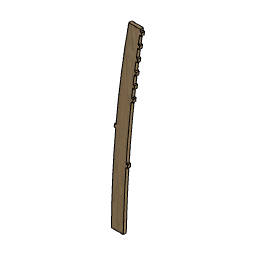
fotur_b (Autodesk Fusion 360 design; units mm, degrees)
Autodesk Fusion 360 part; units mm, degrees
note: some values were not read from the file. Set by a fixed rule: which sketch regions a step uses.
sketch "Sketch1" plane through (0, 0, 0) normal (0, 1, 0) x (1, 0, 0)
  line L0 (0, 0) -> (175, 0)
  line L1 (175, 0) -> (175, -1200)
  line L2 (175, -1200) -> (0, -1200)
  line L3 (0, -1200) -> (0, 0)
  line L4 (0, 0) -> (70, 0)
  line L5 (0, -1200) -> (0, -600)
  arc A0 (70, 0) -> (175, -1200) centre (8172.5, 104.375) ccw
  line L6 (175, -1200) -> (105, -1200)
  arc A1 (0, 0) -> (105, -1200) centre (6634.3619, -24.0871) ccw
  dimension "d1" = 175
  dimension "d2" = 1200
  dimension "d3" = 70
  dimension "d7" = 600
  dimension "d9" = 70
  constraint horizontal L0
  constraint vertical L1
  constraint horizontal L2
  constraint vertical L3
  constraint coincident L0.start L3.end
  constraint perpendicular L3 L4
  constraint perpendicular L2 L5
  constraint perpendicular L1 L6
  measures "d1" distance of L0.start L0.end
  measures "d2" distance of L0.start L2.end
  measures "d3" distance of L0.start L4.end
  measures "d7" distance of L2.end L5.end
  measures "d9" distance of L1.end L6.end
extrude "Extrude1" add sketch "Sketch1" along normal blind 18 contours L0 L2 L3 L4 A0 L6 A1
sketch "Sketch2" plane through (0, 0, 0) normal (0, -1, 0) x (1, 0, 0)
  line L0 (0, 48.1742) -> (0, 0)
  line L1 (0, 0) -> (70, 0)
  arc A0 (175, 1200) -> (70, 0) centre (8172.5, -104.375) ccw
  line L2 (175, 1200) -> (105, 1200)
  arc A1 (105, 1200) -> (0, 48.1742) centre (6634.3619, 24.0871) ccw
  line L3 (172.5991, 1185.1934) -> (181.4831, 1183.7529)
  line L4 (181.4831, 1183.7529) -> (178.282, 1164.0107)
  line L5 (178.282, 1164.0107) -> (169.398, 1165.4512)
  line L6 (172.5991, 1185.1934) -> (169.398, 1165.4512)
  line L7 (150.1002, 1036.8969) -> (159.0061, 1035.5991)
  line L8 (159.0061, 1035.5991) -> (156.1221, 1015.8081)
  line L9 (156.1221, 1015.8081) -> (147.2161, 1017.1059)
  line L10 (139.8807, 962.5964) -> (148.7983, 961.381)
  line L11 (148.7983, 961.381) -> (146.0975, 941.5642)
  line L12 (146.0975, 941.5642) -> (137.18, 942.7795)
  line L13 (130.3495, 888.2053) -> (139.2798, 887.0876)
  line L14 (139.2798, 887.0876) -> (136.796, 867.2424)
  line L15 (136.796, 867.2424) -> (127.8657, 868.3602)
  line L16 (121.5072, 813.729) -> (130.4468, 812.6885)
  line L17 (130.4468, 812.6885) -> (128.1346, 792.8226)
  line L18 (128.1346, 792.8226) -> (119.195, 793.8631)
  line L19 (161.0062, 1111.0952) -> (169.9008, 1109.722)
  line L20 (169.9008, 1109.722) -> (166.8493, 1089.9562)
  line L21 (166.8493, 1089.9562) -> (157.9434, 1091.254)
  dimension "d15" = 15
  dimension "d17" = 9
  dimension "d18" = 20
  dimension "d19" = 9
  dimension "d29" = 9
  dimension "d30" = 20
  dimension "d31" = 9
  dimension "d33" = 9
  dimension "d34" = 20
  dimension "d35" = 9
  dimension "d40" = 55
  dimension "d41" = 9
  dimension "d42" = 20
  dimension "d43" = 9
  dimension "d44" = 55
  dimension "d45" = 9
  dimension "d46" = 20
  dimension "d47" = 9
  dimension "d48" = 55
  dimension "d49" = 9
  dimension "d50" = 20
  dimension "d51" = 9
  constraint perpendicular L3 L4
  constraint perpendicular L4 L5
  constraint coincident A0 L7.start
  constraint perpendicular L7 L8
  constraint perpendicular L8 L9
  constraint coincident A0 L10.start
  constraint perpendicular L10 L11
  constraint perpendicular L11 L12
  constraint coincident A0 L13.start
  constraint perpendicular L13 L14
  constraint perpendicular L14 L15
  constraint coincident A0 L16.start
  constraint perpendicular L16 L17
  constraint perpendicular L17 L18
  constraint coincident A0 L3.start
  constraint coincident A0 L19.start
  constraint perpendicular L19 L20
  measures "d15" distance of A0.start L3.start
  measures "d17" distance of L3.start L3.end
  measures "d18" distance of L3.end L4.end
  measures "d19" distance of L4.end L5.end
  measures "d29" distance of L7.start L7.end
  measures "d30" distance of L7.end L8.end
  measures "d31" distance of L8.end L9.end
  measures "d33" distance of L10.start L10.end
  measures "d34" distance of L10.end L11.end
  measures "d35" distance of L11.end L12.end
  measures "d40" distance of L12.end L13.start
  measures "d41" distance of L13.start L13.end
  measures "d42" distance of L13.end L14.end
  measures "d43" distance of L14.end L15.end
  measures "d44" distance of L15.end L16.start
  measures "d45" distance of L16.start L16.end
  measures "d46" distance of L16.end L17.end
  measures "d47" distance of L17.end L18.end
  measures "d48" distance of L5.end L19.start
  measures "d49" distance of L19.start L19.end
  measures "d50" distance of L19.end L20.end
  measures "d51" distance of L20.end L21.end
extrude "Extrude2" add sketch "Sketch2" against normal blind 18 contours A0 L16 L17 L18 | A0 L3 L4 L5 | A0 L5 L6 | A0 L13 L14 L15 | A0 L19 L20 L21 | A0 L10 L11 L12 | A0 L7 L8 L9
sketch "Sketch3" plane through (0, 0, 0) normal (0, -1, 0) x (1, 0, 0)
  arc A0 (175, 1200) -> (172.5991, 1185.1934) centre (8172.5, -104.375) ccw
  line L0 (175, 1200) -> (105, 1200)
  arc A1 (105, 1200) -> (0, 48.1742) centre (6634.3619, 24.0871) ccw
  line L1 (0, 48.1742) -> (0, 0)
  line L2 (0, 0) -> (70, 0)
  arc A2 (119.2656, 793.8548) -> (70, 0) centre (8172.5, -104.375) ccw
  line L3 (119.2656, 793.8548) -> (128.1346, 792.8226)
  line L4 (128.1346, 792.8226) -> (130.4468, 812.6885)
  line L5 (130.4468, 812.6885) -> (121.5072, 813.729)
  arc A3 (127.9241, 868.3528) -> (121.5072, 813.729) centre (8172.5, -104.375) ccw
  line L6 (127.9241, 868.3528) -> (136.796, 867.2424)
  line L7 (136.796, 867.2424) -> (139.2798, 887.0876)
  line L8 (139.2798, 887.0876) -> (130.3495, 888.2053)
  arc A4 (137.2717, 942.767) -> (130.3495, 888.2053) centre (8172.5, -104.375) ccw
  line L9 (137.2717, 942.767) -> (146.0975, 941.5642)
  line L10 (146.0975, 941.5642) -> (148.7983, 961.381)
  line L11 (148.7983, 961.381) -> (139.8807, 962.5964)
  arc A5 (147.3077, 1017.0926) -> (139.8807, 962.5964) centre (8172.5, -104.375) ccw
  line L12 (147.3077, 1017.0926) -> (156.1221, 1015.8081)
  line L13 (156.1221, 1015.8081) -> (159.0061, 1035.5991)
  line L14 (159.0061, 1035.5991) -> (150.1002, 1036.8969)
  line L15 (158.0195, 1091.2429) -> (166.8493, 1089.9562)
  line L16 (166.8493, 1089.9562) -> (169.9008, 1109.722)
  line L17 (169.9008, 1109.722) -> (161.0062, 1111.0952)
  arc A6 (169.4406, 1165.4443) -> (161.0062, 1111.0952) centre (8172.5, -104.375) ccw
  line L18 (169.4406, 1165.4443) -> (178.282, 1164.0107)
  line L19 (178.282, 1164.0107) -> (181.4831, 1183.7529)
  line L20 (181.4831, 1183.7529) -> (172.5991, 1185.1934)
  line L21 (88.6743, 455.2339) -> (97.6378, 454.4241)
  line L22 (97.6378, 454.4241) -> (95.8383, 434.5052)
  line L23 (95.8383, 434.5052) -> (86.8748, 435.315)
  line L24 (27.8153, 631.4419) -> (18.8644, 632.3806)
  line L25 (18.8644, 632.3806) -> (16.7784, 612.4897)
  line L26 (16.7784, 612.4897) -> (26.7239, 611.4467)
  dimension "d56" = 9
  dimension "d57" = 20
  dimension "d58" = 9
  dimension "d72" = 9
  dimension "d73" = 20
  dimension "d74" = 10
  constraint coincident A2 L21.start
  constraint perpendicular L21 L22
  constraint perpendicular L22 L23
  constraint coincident A1 L24.start
  constraint perpendicular L24 L25
  constraint perpendicular L25 L26
  measures "d56" distance of L21.start L21.end
  measures "d57" distance of L21.end L22.end
  measures "d58" distance of L22.end L23.end
  measures "d72" distance of L24.start L24.end
  measures "d73" distance of L24.end L25.end
  measures "d74" distance of L25.end L26.end
extrude "Extrude3" add sketch "Sketch3" against normal blind 18
sketch "Sketch4" plane through (0, 0, 0) normal (0, -1, 0) x (1, 0, 0)
  arc A0 (175, 1200) -> (172.5991, 1185.1934) centre (8172.5, -104.375) ccw
  line L0 (175, 1200) -> (105, 1200)
  arc A1 (105, 1200) -> (27.8153, 631.4419) centre (6634.3619, 24.0871) ccw
  line L1 (27.8153, 631.4419) -> (18.8644, 632.3806)
  line L2 (18.8644, 632.3806) -> (16.7784, 612.4897)
  line L3 (16.7784, 612.4897) -> (26.0142, 611.5211)
  arc A2 (26.0142, 611.5211) -> (0, 48.1742) centre (6634.3619, 24.0871) ccw
  line L4 (0, 48.1742) -> (0, 0)
  line L5 (0, 0) -> (70, 0)
  arc A3 (87.3174, 435.275) -> (70, 0) centre (8172.5, -104.375) ccw
  line L6 (87.3174, 435.275) -> (95.8383, 434.5052)
  line L7 (95.8383, 434.5052) -> (97.6378, 454.4241)
  line L8 (97.6378, 454.4241) -> (88.6743, 455.2339)
  arc A4 (119.2656, 793.8548) -> (88.6743, 455.2339) centre (8172.5, -104.375) ccw
  line L9 (119.2656, 793.8548) -> (128.1346, 792.8226)
  line L10 (128.1346, 792.8226) -> (130.4468, 812.6885)
  line L11 (130.4468, 812.6885) -> (121.5072, 813.729)
  arc A5 (127.9241, 868.3528) -> (121.5072, 813.729) centre (8172.5, -104.375) ccw
  line L12 (127.9241, 868.3528) -> (136.796, 867.2424)
  line L13 (136.796, 867.2424) -> (139.2798, 887.0876)
  line L14 (139.2798, 887.0876) -> (130.3495, 888.2053)
  arc A6 (137.2717, 942.767) -> (130.3495, 888.2053) centre (8172.5, -104.375) ccw
  line L15 (137.2717, 942.767) -> (146.0975, 941.5642)
  line L16 (146.0975, 941.5642) -> (148.7983, 961.381)
  line L17 (148.7983, 961.381) -> (139.8807, 962.5964)
  arc A7 (147.3077, 1017.0926) -> (139.8807, 962.5964) centre (8172.5, -104.375) ccw
  line L18 (147.3077, 1017.0926) -> (156.1221, 1015.8081)
  line L19 (156.1221, 1015.8081) -> (159.0061, 1035.5991)
  line L20 (159.0061, 1035.5991) -> (150.1002, 1036.8969)
  line L21 (158.0195, 1091.2429) -> (166.8493, 1089.9562)
  line L22 (166.8493, 1089.9562) -> (169.9008, 1109.722)
  line L23 (169.9008, 1109.722) -> (161.0062, 1111.0952)
  arc A8 (169.4406, 1165.4443) -> (161.0062, 1111.0952) centre (8172.5, -104.375) ccw
  line L24 (169.4406, 1165.4443) -> (178.282, 1164.0107)
  line L25 (178.282, 1164.0107) -> (181.4831, 1183.7529)
  line L26 (181.4831, 1183.7529) -> (172.5991, 1185.1934)
  line L27 (0, 0) -> (0, 80)
  line L28 (0, 80) -> (71.4256, 80)
  line L29 (71.4256, 80) -> (70, 0)
  line L30 (70, 0) -> (0, 0)
  arc A9 (158.0195, 1091.2429) -> (150.1002, 1036.8969) centre (8172.5, -104.375) ccw
  dimension "d76" = 80
  constraint coincident L4.end L5.start
  constraint parallel L4 L27
  constraint coincident A3 L28.end
  constraint perpendicular L27 L28
  constraint coincident L5.end A3.end
  measures "d76" distance of L4.end L27.end
extrude "Extrude4" cut sketch "Sketch4" against normal blind 18 contours A2 L4 L5 A3 L27 L28 L30
equation "d1 = heildarbreidd"
equation "d2 = haed_fots"
equation "d3 = breidd_fots"
equation "breidd_fots = 70 mm"
equation "haed_fots = 1200 mm"
equation "heildarbreidd = 175 mm"
equation "d7 = haed_fots / 2"
equation "d9 = breidd_fots"
equation "t = 18 mm"
equation "d11 = t"
equation "nibba_bil = 15 mm"
equation "nibba_breidd = 20 mm"
equation "d15 = nibba_bil"
equation "nibba_lengd = 9 mm"
equation "d17 = nibba_lengd"
equation "d18 = nibba_breidd"
equation "d19 = nibba_lengd"
equation "d20 = -t"
equation "biti_bil = 25 mm"
equation "d29 = nibba_lengd"
equation "d30 = nibba_breidd"
equation "d31 = nibba_lengd"
equation "d33 = nibba_lengd"
equation "d34 = nibba_breidd"
equation "d35 = nibba_lengd"
equation "d40 = 2 * nibba_bil + biti_bil"
equation "d41 = nibba_lengd"
equation "d42 = nibba_breidd"
equation "d43 = nibba_lengd"
equation "d44 = 2 * nibba_bil + biti_bil"
equation "d45 = nibba_lengd"
equation "d46 = nibba_breidd"
equation "d47 = nibba_lengd"
equation "d48 = 2 * nibba_bil + biti_bil"
equation "d49 = nibba_lengd"
equation "d50 = nibba_breidd"
equation "plata_þykkt = 50 mm"
equation "bil_fremri_stod = 95 mm"
equation "d56 = nibba_lengd"
equation "d57 = nibba_breidd"
equation "d58 = nibba_lengd"
equation "d59 = -t"
equation "breidd_fots2 = 90 mm"
equation "bil_support1 = 140 mm"
equation "d72 = nibba_lengd"
equation "d73 = nibba_breidd"
equation "d74 = nibba_lengd + 1 mm"
equation "bil_support2 = 165 mm"
